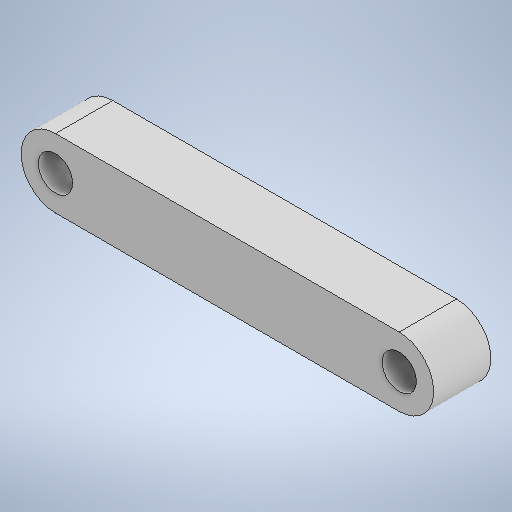
# Autodesk Inventor part: SuspensionFrame
Saved by Autodesk Inventor 2025.2 (Build 292293000, 293)
## iProperties
Created: 2025-01-05
Part Number: SuspensionFrame
Material: 일반
Document SubType Name: Modeling
Designer: SEON
Density: 1 g/cm^3
Appearance: 기본값
Author: SEON
Autodesk Inventor part; units mm, degrees
ref_plane "YZ Plane" through (0, 0, 0) normal (1, 0, 0) x (0, 1, 0)
ref_plane "XZ Plane" through (0, 0, 0) normal (0, 1, 0) x (-1, 0, 0)
ref_plane "XY Plane" through (0, 0, 0) normal (0, 0, 1) x (1, 0, 0)
sketch "스케치1" plane through (0, 0, 0) normal (0, 0, 1) x (1, 0, 0)
  line L0 (0, 0) -> (30, 0) construction
  line L1 (0, -3) -> (30, -3)
  line L2 (30, 3) -> (0, 3)
  arc A0 (0, 3) -> (0, -3) centre (0, 0) ccw
  arc A1 (30, -3) -> (30, 3) centre (30, 0) ccw
  circle A2 centre (0, 0) radius 1.5
  circle A3 centre (30, 0) radius 1.5
  point P0 (15, 0)
  dimension "d0" = 6
  dimension "d1" = 3
  dimension "d2" = 3
  dimension "d3" = 30
  constraints: 8 end point, 4 centre point, 4 point on circle, 4 tangent, 2 coincident, 1 horizontal, 1 midpoint, 1 parallel
  measures "d0" distance between parallel lines of L1 L2
  measures "d1" diameter of A2
  measures "d2" diameter of A3
  measures "d3" distance of L0.start L0.end
extrude "돌출1" add sketch "스케치1" along normal blind 5
